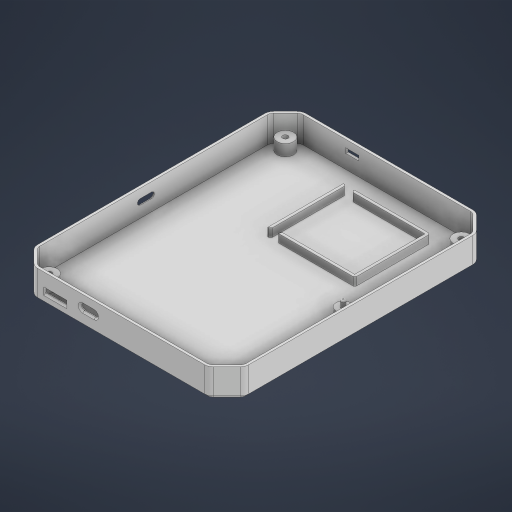
# Autodesk Inventor part: keypad_layout
Saved by Autodesk Inventor 2024 (Build 280153000, 153)
## iProperties
Created: 2023-11-21
Part Number: keypad_layout
Material: Generic
Document SubType Name: Modeling
Designer: minekuba
Density: 1 g/cm^3
Appearance: Default
Author: minekuba
Autodesk Inventor part; units mm, degrees
ref_plane "YZ Plane" through (0, 0, 0) normal (1, 0, 0) x (0, 1, 0)
ref_plane "XZ Plane" through (0, 0, 0) normal (0, 1, 0) x (-1, 0, 0)
ref_plane "XY Plane" through (0, 0, 0) normal (0, 0, 1) x (1, 0, 0)
sketch "Sketch1" plane through (0, 0, 0) normal (0, 1, 0) x (-1, 0, 0)
  line L0 (51.2574, 80) -> (-51.2574, 80)
  line L1 (-62.5, 68.7574) -> (-62.5, -68.7574)
  line L2 (-51.2574, -80) -> (51.2574, -80)
  line L3 (62.5, 80) -> (-62.5, -80) construction
  line L4 (-62.5, 80) -> (62.5, -80) construction
  line L5 (60.6213, 71.8787) -> (53.3787, 79.1213)
  line L6 (60.6213, -71.8787) -> (53.3787, -79.1213)
  line L7 (-53.3787, -79.1213) -> (-61.6213, -70.8787)
  line L8 (-53.3787, 79.1213) -> (-61.6213, 70.8787)
  arc A0 (61.5, 69.7574) -> (60.6213, 71.8787) centre (58.5, 69.7574) ccw
  arc A1 (53.3787, 79.1213) -> (51.2574, 80) centre (51.2574, 77) ccw
  arc A2 (-51.2574, 80) -> (-53.3787, 79.1213) centre (-51.2574, 77) ccw
  arc A3 (-61.6213, 70.8787) -> (-62.5, 68.7574) centre (-59.5, 68.7574) ccw
  arc A4 (-62.5, -68.7574) -> (-61.6213, -70.8787) centre (-59.5, -68.7574) ccw
  arc A5 (-53.3787, -79.1213) -> (-51.2574, -80) centre (-51.2574, -77) ccw
  arc A6 (60.6213, -71.8787) -> (61.5, -69.7574) centre (58.5, -69.7574) ccw
  arc A7 (51.2574, -80) -> (53.3787, -79.1213) centre (51.2574, -77) ccw
  line L9 (60.5, 42) -> (56.5, 42)
  line L10 (55.5, 41) -> (55.5, 23)
  line L11 (56.5, 22) -> (60.5, 22)
  line L12 (61.5, -69.7574) -> (61.5, 21)
  line L13 (61.5, 43) -> (61.5, 69.7574)
  arc A8 (60.5, 42) -> (61.5, 43) centre (60.5, 43) ccw
  arc A9 (56.5, 42) -> (55.5, 41) centre (56.5, 41) ccw
  arc A10 (55.5, 23) -> (56.5, 22) centre (56.5, 23) ccw
  arc A11 (61.5, 21) -> (60.5, 22) centre (60.5, 21) ccw
  circle A12 centre (54, 72.5) radius 1.65
  line L14 (67, 0) -> (-74, 0) construction
  line L15 (54, 72.5) -> (57, 75.5) construction
  circle A13 centre (54, -72.5) radius 1.65
  line L16 (0, 82) -> (0, -121) construction
  circle A14 centre (-54, 72.5) radius 1.65
  circle A15 centre (-54, -72.5) radius 1.65
  circle A16 centre (-54, 0) radius 1.65
  point P0 (0, 0)
  point P1 (62.5, 70)
  point P2 (52.5, 80)
  point P3 (62.5, -70)
  point P4 (52.5, -80)
  point P5 (-52.5, -80)
  point P6 (-62.5, -70)
  point P7 (-52.5, 80)
  point P8 (-62.5, 70)
  point P9 (55.5, 22)
  point P10 (61.5, 22)
  point P11 (58.5, 42)
  point P12 (58.5, 22)
  dimension "d0" = 125
  dimension "d1" = 160
  dimension "d2" = 10
  dimension "d3" = 10
  dimension "d4" = 10
  dimension "d5" = 10
  dimension "d6" = 10
  dimension "d7" = 10
  dimension "d8" = 10
  dimension "d9" = 10
  dimension "d10" = 3
  dimension "d11" = 38
  dimension "d12" = 102
  dimension "d13" = 6
  dimension "d14" = 1
  dimension "d15" = 3.3
  dimension "d17" = 3
  constraints: 34 end point, 26 tangent, 25 point on line, 24 point on circle, 17 centre point, 11 equal radius, 5 midpoint, 4 parallel, 3 horizontal, 3 perpendicular, 3 symmetric about line, 1 line through centre, 1 vertical, 3 other
  measures "d0" distance of L4.end L3.end
  measures "d1" distance of L3.end L4.start
  measures "d2" distance of point (62.5, 70) L3.start
  measures "d3" distance of point (52.5, 80) L3.start
  measures "d4" distance of point (62.5, -70) L4.end
  measures "d5" distance of point (52.5, -80) L4.end
  measures "d6" distance of point (-52.5, -80) L3.end
  measures "d7" distance of point (-62.5, -70) L3.end
  measures "d8" distance of point (-52.5, 80) L4.start
  measures "d9" distance of point (-62.5, 70) L4.start
  measures "d10" radius of A0
  measures "d11" distance from line of L0 point (58.5, 42)
  measures "d12" distance from line of L2 point (58.5, 22)
  measures "d13" distance of point (55.5, 22) point (61.5, 22)
  measures "d14" radius of A8
  measures "d15" diameter of A12
  measures "d17" horizontal distance of L15.start L15.end
sketch "Sketch2" plane through (0, 0, 0) normal (0, 1, 0) x (-1, 0, 0)
  line L0 (60.6213, -71.8787) -> (53.3787, -79.1213) construction
  arc A0 (51.2574, -80) -> (53.3787, -79.1213) centre (51.2574, -77) ccw construction
  arc A1 (60.6213, -71.8787) -> (61.5, -69.7574) centre (58.5, -69.7574) ccw construction
  line L1 (61.5, -69.7574) -> (61.5, 21) construction
  arc A2 (61.5, 21) -> (60.5, 22) centre (60.5, 21) ccw construction
  line L2 (56.5, 22) -> (60.5, 22) construction
  arc A3 (55.5, 23) -> (56.5, 22) centre (56.5, 23) ccw construction
  line L3 (55.5, 41) -> (55.5, 23) construction
  arc A4 (56.5, 42) -> (55.5, 41) centre (56.5, 41) ccw construction
  arc A5 (60.5, 42) -> (61.5, 43) centre (60.5, 43) ccw construction
  line L4 (61.5, 43) -> (61.5, 69.7574) construction
  arc A6 (61.5, 69.7574) -> (60.6213, 71.8787) centre (58.5, 69.7574) ccw construction
  line L5 (60.6213, 71.8787) -> (53.3787, 79.1213) construction
  arc A7 (53.3787, 79.1213) -> (51.2574, 80) centre (51.2574, 77) ccw construction
  line L6 (51.2574, 80) -> (-51.2574, 80) construction
  arc A8 (-51.2574, 80) -> (-53.3787, 79.1213) centre (-51.2574, 77) ccw construction
  line L7 (-53.3787, 79.1213) -> (-61.6213, 70.8787) construction
  arc A9 (-61.6213, 70.8787) -> (-62.5, 68.7574) centre (-59.5, 68.7574) ccw construction
  line L8 (-62.5, 68.7574) -> (-62.5, -68.7574) construction
  arc A10 (-62.5, -68.7574) -> (-61.6213, -70.8787) centre (-59.5, -68.7574) ccw construction
  line L9 (-53.3787, -79.1213) -> (-61.6213, -70.8787) construction
  arc A11 (-53.3787, -79.1213) -> (-51.2574, -80) centre (-51.2574, -77) ccw construction
  line L10 (-51.2574, -80) -> (51.2574, -80) construction
  line L11 (60.5, 42) -> (56.5, 42) construction
  line L12 (53.9444, 79.687) -> (61.187, 72.4444)
  arc A12 (62.3, 69.7574) -> (61.187, 72.4444) centre (58.5, 69.7574) ccw
  line L13 (62.3, 69.7574) -> (62.3, 43)
  line L14 (62.3, 21) -> (62.3, -69.7574)
  arc A13 (61.187, -72.4444) -> (62.3, -69.7574) centre (58.5, -69.7574) ccw
  line L15 (61.187, -72.4444) -> (53.9444, -79.687)
  arc A14 (51.2574, -80.8) -> (53.9444, -79.687) centre (51.2574, -77) ccw
  line L16 (51.2574, -80.8) -> (-51.2574, -80.8)
  arc A15 (-53.9444, -79.687) -> (-51.2574, -80.8) centre (-51.2574, -77) ccw
  line L17 (-53.9444, -79.687) -> (-62.187, -71.4444)
  arc A16 (-63.3, -68.7574) -> (-62.187, -71.4444) centre (-59.5, -68.7574) ccw
  line L18 (-63.3, -68.7574) -> (-63.3, 68.7574)
  arc A17 (-62.187, 71.4444) -> (-63.3, 68.7574) centre (-59.5, 68.7574) ccw
  line L19 (-62.187, 71.4444) -> (-53.9444, 79.687)
  arc A18 (-51.2574, 80.8) -> (-53.9444, 79.687) centre (-51.2574, 77) ccw
  line L20 (-51.2574, 80.8) -> (51.2574, 80.8)
  arc A19 (53.9444, 79.687) -> (51.2574, 80.8) centre (51.2574, 77) ccw
  line L21 (62.3, 43) -> (62.3, 21)
  line L22 (63.8, 43) -> (63.8, 69.7574)
  arc A20 (63.8, 69.7574) -> (62.2477, 73.505) centre (58.5, 69.7574) ccw
  line L23 (62.2477, 73.505) -> (55.005, 80.7477)
  arc A21 (55.005, 80.7477) -> (51.2574, 82.3) centre (51.2574, 77) ccw
  line L24 (51.2574, 82.3) -> (-51.2574, 82.3)
  arc A22 (-51.2574, 82.3) -> (-55.005, 80.7477) centre (-51.2574, 77) ccw
  line L25 (-55.005, 80.7477) -> (-63.2477, 72.505)
  arc A23 (-63.2477, 72.505) -> (-64.8, 68.7574) centre (-59.5, 68.7574) ccw
  line L26 (-64.8, 68.7574) -> (-64.8, -68.7574)
  arc A24 (-64.8, -68.7574) -> (-63.2477, -72.505) centre (-59.5, -68.7574) ccw
  line L27 (-63.2477, -72.505) -> (-55.005, -80.7477)
  arc A25 (-55.005, -80.7477) -> (-51.2574, -82.3) centre (-51.2574, -77) ccw
  line L28 (-51.2574, -82.3) -> (51.2574, -82.3)
  arc A26 (51.2574, -82.3) -> (55.005, -80.7477) centre (51.2574, -77) ccw
  line L29 (55.005, -80.7477) -> (62.2477, -73.505)
  arc A27 (62.2477, -73.505) -> (63.8, -69.7574) centre (58.5, -69.7574) ccw
  line L30 (63.8, -69.7574) -> (63.8, 21)
  line L31 (63.8, 21) -> (63.8, 43)
  point P0 (0, 0)
  dimension "d18" = 0.8
  dimension "d19" = 1.5
  constraints: 40 end point, 32 point on circle, 16 centre point, 1 vertical, 32 other
  measures "d18" distance between parallel lines of L5 L12
  measures "d19" distance between parallel lines of L13 L22
extrude "Extrusion1" add sketch "Sketch2" along normal blind 1.5 contours L12 A12 L13 L21 L14 A13 L15 A14 L16 A15 L17 A16 L18 A17 L19 A18 L20 A19 | L31 L30 A27 L29 A26 L28 A25 L27 A24 L26 A23 L25 A22 L24 A21 L23 A20 L22
sketch "Sketch4" plane through (0, 1.5, 0) normal (0, 1, 0) x (1, 0, 0)
  arc A0 (-63.8, -69.7574) -> (-62.2477, -73.505) centre (-58.5, -69.7574) ccw projected
  line L0 (-62.2477, -73.505) -> (-55.005, -80.7477) projected
  arc A1 (-55.005, -80.7477) -> (-51.2574, -82.3) centre (-51.2574, -77) ccw projected
  line L1 (-51.2574, -82.3) -> (51.2574, -82.3) projected
  arc A2 (51.2574, -82.3) -> (55.005, -80.7477) centre (51.2574, -77) ccw projected
  line L2 (55.005, -80.7477) -> (63.2477, -72.505) projected
  arc A3 (63.2477, -72.505) -> (64.8, -68.7574) centre (59.5, -68.7574) ccw projected
  line L3 (64.8, -68.7574) -> (64.8, 68.7574) projected
  arc A4 (64.8, 68.7574) -> (63.2477, 72.505) centre (59.5, 68.7574) ccw projected
  line L4 (63.2477, 72.505) -> (55.005, 80.7477) projected
  arc A5 (55.005, 80.7477) -> (51.2574, 82.3) centre (51.2574, 77) ccw projected
  line L5 (51.2574, 82.3) -> (-51.2574, 82.3) projected
  arc A6 (-51.2574, 82.3) -> (-55.005, 80.7477) centre (-51.2574, 77) ccw projected
  line L6 (-55.005, 80.7477) -> (-62.2477, 73.505) projected
  arc A7 (-62.2477, 73.505) -> (-63.8, 69.7574) centre (-58.5, 69.7574) ccw projected
  line L7 (-63.8, 69.7574) -> (-63.8, -69.7574) projected
  line L8 (51.2574, -80.8) -> (-51.2574, -80.8)
  arc A8 (-53.9444, -79.687) -> (-51.2574, -80.8) centre (-51.2574, -77) ccw
  line L9 (-53.9444, -79.687) -> (-61.187, -72.4444)
  arc A9 (-62.3, -69.7574) -> (-61.187, -72.4444) centre (-58.5, -69.7574) ccw
  line L10 (-62.3, -69.7574) -> (-62.3, 69.7574)
  arc A10 (-61.187, 72.4444) -> (-62.3, 69.7574) centre (-58.5, 69.7574) ccw
  line L11 (-61.187, 72.4444) -> (-53.9444, 79.687)
  arc A11 (-51.2574, 80.8) -> (-53.9444, 79.687) centre (-51.2574, 77) ccw
  line L12 (-51.2574, 80.8) -> (51.2574, 80.8)
  arc A12 (53.9444, 79.687) -> (51.2574, 80.8) centre (51.2574, 77) ccw
  line L13 (53.9444, 79.687) -> (62.187, 71.4444)
  arc A13 (63.3, 68.7574) -> (62.187, 71.4444) centre (59.5, 68.7574) ccw
  line L14 (63.3, 68.7574) -> (63.3, -68.7574)
  arc A14 (62.187, -71.4444) -> (63.3, -68.7574) centre (59.5, -68.7574) ccw
  line L15 (62.187, -71.4444) -> (53.9444, -79.687)
  arc A15 (51.2574, -80.8) -> (53.9444, -79.687) centre (51.2574, -77) ccw
  point P0 (0, 0)
  dimension "d22" = 1.5
  constraints: 16 end point, 16 point on circle, 8 centre point, 15 other
  measures "d22" distance between parallel lines of L1 L8
extrude "Extrusion2" add sketch "Sketch4" along normal blind 16
sketch "Sketch5" plane through (0, 1.5, 0) normal (0, 1, 0) x (1, 0, 0)
  circle A0 centre (-54, -72.5) radius 1.65 projected
  circle A1 centre (-54, 72.5) radius 1.65 projected
  circle A2 centre (54, 72.5) radius 1.65 projected
  circle A3 centre (54, 0) radius 1.65 construction
  circle A4 centre (54, -72.5) radius 1.65 projected
  circle A5 centre (-54, -72.5) radius 5.0426
  line L0 (-53.9444, -79.687) -> (-61.187, -72.4444) projected
  circle A6 centre (-54, 72.5) radius 5.0426
  line L1 (-61.187, 72.4444) -> (-53.9444, 79.687) projected
  circle A7 centre (54, 72.5) radius 5.0426
  line L2 (62.187, 71.4444) -> (53.9444, 79.687) projected
  circle A8 centre (54, 0) radius 4.4425
  circle A9 centre (54, -72.5) radius 5.0426
  line L3 (62.187, -71.4444) -> (53.9444, -79.687) projected
  point P0 (0, 0)
  dimension "d25" = 8.885
  constraints: 5 centre point, 5 coincident, 4 tangent
  measures "d25" diameter of A8
extrude "Extrusion3" add sketch "Sketch5" along normal blind 7
sketch "Sketch6" plane through (51.2574, 0, -82.3) normal (0, 0, -1) x (-1, 0, 0)
  line L0 (115.0574, 0) -> (115.0574, 17.5) projected
  line L1 (0, 0) -> (102.5147, 0) projected
  line L2 (76.5574, 13) -> (68.5574, 13)
  line L3 (68.5574, 13) -> (68.5574, 10)
  line L4 (68.5574, 10) -> (76.5574, 10)
  line L5 (76.5574, 10) -> (76.5574, 13)
  point P0 (51.2574, 0)
  point P1 (76.5574, 11.5)
  dimension "d28" = 10
  dimension "d29" = 38.5
  dimension "d30" = 8
  dimension "d31" = 3
  constraints: 8 end point, 2 parallel, 1 horizontal, 1 midpoint, 1 perpendicular
  measures "d28" distance between parallel lines of L1 L4
  measures "d29" distance from line of L0 point (76.557, 11.5)
  measures "d30" distance of L2.start L2.end
  measures "d31" distance of L2.end L3.end
extrude "Extrusion4" cut sketch "Sketch6" against normal blind 5
sketch "Sketch7" plane through (0, 1.5, 0) normal (0, 1, 0) x (1, 0, 0)
  line L0 (-6.7, 22.8) -> (38.3, 22.8)
  line L1 (38.3, 22.8) -> (38.3, 65.8)
  line L2 (38.3, 65.8) -> (-6.7, 65.8)
  line L3 (-11.7, 65.8) -> (-11.7, 22.8)
  line L4 (-51.2574, 80.8) -> (51.2574, 80.8) projected
  line L5 (63.3, 68.7574) -> (63.3, -68.7574) projected
  line L6 (40, 21.1) -> (40, 67.5)
  line L7 (-13.4, 67.5) -> (-13.4, 21.1)
  line L8 (-11.7, 22.8) -> (-11.7, 21.1)
  line L9 (-6.7, 21.1) -> (-6.7, 22.8)
  line L10 (-13.4, 21.1) -> (-11.7, 21.1)
  line L11 (-6.7, 21.1) -> (40, 21.1)
  line L12 (-11.7, 65.8) -> (-11.7, 67.5)
  line L13 (-6.7, 65.8) -> (-6.7, 67.5)
  line L14 (40, 67.5) -> (-6.7, 67.5)
  line L15 (-11.7, 67.5) -> (-13.4, 67.5)
  point P0 (0, 0)
  point P1 (-6.7, 66.65)
  dimension "d34" = 50
  dimension "d35" = 43
  dimension "d36" = 15
  dimension "d37" = 25
  dimension "d40" = 5
  dimension "d41" = 5
  constraints: 28 end point, 10 perpendicular, 7 parallel, 1 horizontal, 1 midpoint
  measures "d34" distance of L3.start L1.end
  measures "d35" distance of L1.end L0.end
  measures "d36" distance between parallel lines of L4 L2
  measures "d37" distance between parallel lines of L5 L1
  measures "d40" distance between parallel lines of L9 L8
  measures "d41" distance from line of point (-6.7, 66.65) L12
extrude "Extrusion5" add sketch "Sketch7" along normal blind 5
sketch "Sketch8" plane through (-13.4, 1.5, -21.1) normal (0, 0, 1) x (1, 0, 0)
  point P0 (13.4, -1.5)
chamfer "Chamfer1" distance 2 angle 45 16 edges at (0, 0, -82.3) (-53.2856, 0, -81.8966) (-58.6263, 0, -77.1263) (-63.3966, 0, -71.7856) (-63.8, 0, 0) (-63.3966, 0, 71.7856) (-58.6263, 0, 77.1263) (-53.2856, 0, 81.8966) (0, 0, 82.3) (53.2856, 0, 81.8966) (59.1263, 0, 76.6263) (64.3966, 0, 70.7856) (64.8, 0, 0) (64.3966, 0, -70.7856) (59.1263, 0, -76.6263) (53.2856, 0, -81.8966)
chamfer "Chamfer2" distance 1 angle 45 6 edges at (40, 4, -21.1) (40, 4, -67.5) (-11.7, 4, -67.5) (-11.7, 4, -21.1) (-6.7, 4, -65.8) (-6.7, 4, -22.8)
sketch "Sketch10" plane through (54, 8.5, 0) normal (0, 1, 0) x (1, 0, 0)
  circle A0 centre (0, 0) radius 4.4425 projected
  circle A1 centre (0, 0) radius 1.4
  point P0 (-54, 0)
  dimension "d81" = 2.8
  constraints: 1 centre point, 1 coincident
  measures "d81" diameter of A1
extrude "Extrusion6" add sketch "Sketch10" along normal blind 4 contours A1
fillet "Fillet1" radius 1 1 edges at (52.6, 12.5, 0)
sketch "Sketch11" plane through (-63.8, 17.5, -69.7574) normal (-1, 0, 0) x (0, 0, 1)
  line L0 (139.5147, -15.5) -> (0, -15.5) projected
  line L1 (139.5147, -15.5) -> (139.5147, 0) projected
  line L2 (0, 0) -> (139.5147, 0) projected
  line L3 (0, -15.5) -> (0, 0) projected
  line L4 (0, -17.5) -> (139.5147, -17.5) projected
  line L5 (71.0574, -7.25) -> (78.0574, -7.25) construction
  line L6 (71.0574, -9) -> (78.0574, -9)
  line L7 (78.0574, -5.5) -> (71.0574, -5.5)
  arc A0 (71.0574, -5.5) -> (71.0574, -9) centre (71.0574, -7.25) ccw
  arc A1 (78.0574, -9) -> (78.0574, -5.5) centre (78.0574, -7.25) ccw
  line L8 (152.0574, -15.5) -> (152.0574, 0) projected
  point P0 (69.7574, -17.5)
  point P1 (74.5574, -7.25)
  point P2 (69.7574, -17.5)
  point P3 (74.5574, -9)
  dimension "d52" = 1.75
  dimension "d53" = 7
  dimension "d78" = 74
  dimension "d79" = 8.5
  constraints: 8 end point, 4 point on circle, 4 tangent, 3 midpoint, 2 centre point, 2 parallel
  measures "d52" radius of A1
  measures "d53" distance of L5.start L5.end
  measures "d78" distance from line of L8 L5.end
  measures "d79" distance from line of L4 point (74.557, -9)
extrude "Extrusion7" cut sketch "Sketch11" against normal blind 4 contours A0 L7 A1 L6
chamfer "Chamfer3" distance 1 angle 45 4 edges at (-63.8, 12, 4.8) (-63.8, 10.25, 10.05) (-63.8, 8.5, 4.8) (-63.8, 10.25, -0.45)
sketch "Sketch12" plane through (-51.2574, 17.5, 82.3) normal (0, 0, 1) x (1, 0, 0)
  line L0 (0, -17.5) -> (102.5147, -17.5) projected
  line L1 (-12.5426, -15.5) -> (-12.5426, 0) projected
  line L2 (3.9574, -9) -> (17.9574, -9)
  line L3 (17.9574, -9) -> (17.9574, -11.5)
  line L4 (17.9574, -11.5) -> (3.9574, -11.5)
  line L5 (3.9574, -11.5) -> (3.9574, -9)
  point P0 (51.2574, -17.5)
  dimension "d59" = 16.5
  dimension "d61" = 8.5
  dimension "d62" = 14
  dimension "d63" = 2.5
  constraints: 8 end point, 2 parallel, 1 horizontal, 1 perpendicular
  measures "d59" distance between parallel lines of L1 L5
  measures "d61" distance between parallel lines of L0 L2
  measures "d62" distance of L2.start L2.end
  measures "d63" distance of L2.end L3.end
extrude "Extrusion8" cut sketch "Sketch12" against normal blind 4
chamfer "Chamfer5" distance 1 angle 45 2 edges at (-40.3, 6, 82.3) (-40.3, 8.5, 82.3)
sketch "Sketch14" plane through (-51.2574, 17.5, 82.3) normal (0, 0, 1) x (1, 0, 0)
  line L0 (-12.5426, -15.5) -> (-12.5426, 0) projected
  line L1 (0, -17.5) -> (102.5147, -17.5) projected
  line L2 (27.7074, -7.25) -> (34.7074, -7.25) construction
  line L3 (27.7074, -5.5) -> (34.7074, -5.5)
  line L4 (34.7074, -9) -> (27.7074, -9)
  arc A0 (27.7074, -5.5) -> (27.7074, -9) centre (27.7074, -7.25) ccw
  arc A1 (34.7074, -9) -> (34.7074, -5.5) centre (34.7074, -7.25) ccw
  point P0 (51.2574, -17.5)
  point P1 (31.2074, -7.25)
  point P2 (25.9574, -7.25)
  dimension "d66" = 38.5
  dimension "d67" = 8.5
  dimension "d68" = 1.75
  dimension "d69" = 7
  constraints: 8 end point, 5 point on circle, 4 tangent, 2 centre point, 1 horizontal, 1 midpoint, 1 parallel
  measures "d66" distance from line of point (25.957, -7.25) L0
  measures "d67" distance between parallel lines of L1 L4
  measures "d68" radius of A1
  measures "d69" distance of L2.start L2.end
extrude "Extrusion9" cut sketch "Sketch14" against normal blind 4
chamfer "Chamfer4" distance 1 angle 45 4 edges at (-20.05, 12, 82.3) (-14.8, 10.25, 82.3) (-20.05, 8.5, 82.3) (-25.3, 10.25, 82.3)
equation "\"d3\" = d2"
equation "\"d4\" = d2"
equation "\"d5\" = d4"
equation "\"d6\" = d2"
equation "\"d7\" = d6"
equation "\"d8\" = d2"
equation "\"d9\" = d8"
body "Solid1"
